Autodesk Fusion 360 part; units mm, degrees
(part 2 of 2)
sketch "Sketch8" plane through (0, 0, -25.2) normal (0, 0, -1) x (1, 0, 0)
  circle A0 centre (107.1093, 9.6234) radius 1.85
  circle A1 centre (13.8605, 220.7337) radius 1.85
  circle A2 centre (13.8605, 111.1767) radius 1.85
  circle A3 centre (13.8605, 9.6234) radius 1.85
  circle A4 centre (107.1093, 220.7337) radius 1.85
  circle A5 centre (106.1086, 111.1767) radius 1.85
  line L0 (118.8791, -2.2165) -> (118.8791, 232.5835)
  line L1 (118.8791, 232.5835) -> (2.0791, 232.5835)
  line L2 (2.0791, 232.5835) -> (2.0791, -2.2165)
  line L3 (2.0791, -2.2165) -> (118.8791, -2.2165)
  circle A6 centre (107.1093, 9.6234) radius 4.65
  circle A7 centre (106.1086, 111.1767) radius 4.65
  circle A8 centre (107.1093, 220.7337) radius 4.65
  line L4 (60.4791, 232.5835) -> (60.4791, -2.2165) construction
  circle A9 centre (13.8605, 111.1767) radius 4.65
  circle A10 centre (13.8605, 220.7337) radius 4.65
  circle A11 centre (13.8605, 9.6234) radius 4.65
  circle A12 centre (107.1093, 220.7337) radius 6.65
  circle A13 centre (13.8605, 220.7337) radius 6.65
  circle A14 centre (106.1086, 111.1767) radius 6.65
  circle A15 centre (13.8605, 111.1767) radius 6.65
  circle A16 centre (13.8605, 9.6234) radius 6.65
  circle A17 centre (107.1093, 9.6234) radius 6.65
  circle A18 centre (13.8605, 9.6234) radius 1.85
  circle A19 centre (13.8605, 111.1767) radius 1.85
  circle A20 centre (107.1093, 220.7337) radius 1.85
  circle A21 centre (106.1086, 111.1767) radius 1.85
  circle A22 centre (13.8605, 220.7337) radius 1.85
  circle A23 centre (107.1093, 9.6234) radius 1.85
  line L5 (111.4791, 5.1835) -> (9.4791, 5.1835)
  line L6 (9.4791, 5.1835) -> (9.4791, 225.1835)
  line L7 (9.4791, 225.1835) -> (111.4791, 225.1835)
  line L8 (111.4791, 225.1835) -> (111.4791, 5.1835)
  line L9 (9.4791, 117.8267) -> (13.8605, 117.8267)
  line L10 (13.8605, 117.8267) -> (13.8605, 104.5267) construction
  line L11 (13.8605, 104.5267) -> (9.4791, 104.5267)
  line L12 (9.4791, 104.5267) -> (9.4791, 117.8267)
  line L13 (111.4791, 117.8267) -> (106.1086, 117.8267)
  line L14 (106.1086, 117.8267) -> (106.1086, 104.5267) construction
  line L15 (106.1086, 104.5267) -> (111.4791, 104.5267)
  line L16 (111.4791, 104.5267) -> (111.4791, 117.8267)
  dimension "d128" = 9.3
  dimension "d129" = 9.3
  dimension "d130" = 9.3
  dimension "d131" = 9.3
  dimension "d132" = 9.3
  dimension "d133" = 9.3
  dimension "d170" = 2
  dimension "d171" = 2
  dimension "d172" = 2
  dimension "d173" = 2
  dimension "d174" = 2
  dimension "d175" = 2
  constraint concentric A0 A6
  constraint concentric A5 A7
  constraint concentric A4 A8
  constraint midpoint L1 L4.start
  constraint midpoint L3 L4.end
  constraint concentric A2 A9
  constraint concentric A1 A10
  constraint concentric A3 A11
  constraint horizontal L9
  constraint vertical L10
  constraint horizontal L11
  constraint vertical L12
  constraint coincident A15 L10.end
  constraint coincident L6 L9.start
  constraint tangent A15 L9
  constraint tangent A15 L11
  constraint horizontal L13
  constraint vertical L14
  constraint horizontal L15
  constraint vertical L16
  constraint coincident A14 L14.end
  constraint coincident L8 L13.start
  constraint tangent A14 L15
  constraint tangent A14 L13
  measures "d128" diameter of A6
  measures "d129" diameter of A7
  measures "d130" diameter of A8
  measures "d131" diameter of A9
  measures "d132" diameter of A10
  measures "d133" diameter of A11
extrude "Extrude17" add sketch "Sketch8" against normal up to surface (6 mm away) contours A6 L8 | A6 A17 L5 L8 | A6 L5 L8 | A6 A17 L5 L8 | A6 L5 L8 | A6 L5 | A14 L8 L15 L16 | A11 A16 L5 L6 | A11 A16 L5 L6 | A14 L8 L16 | A14 L8 L16 | A11 L5 L6 | A11 L5 | A14 L8 L13 L16 | A11 L6 | A15 L6 L11 L12 | A11 L5 L6 | A9 A15 L6 L12 | A9 A15 L6 L12 | A8 A12 L7 L8 | A8 A12 L7 L8 | A15 L6 L9 L12 | A9 L6 L12 | A9 L6 L12 | A8 L8 | A8 L7 L8 | A10 A13 L6 L7 | A10 A13 L6 L7 | A8 L7 | A8 L7 L8 | A10 L7 | A10 L6 L7 | A10 L6 | A10 L6 L7 | A7 bodies 2
extrude "Extrude13" cut sketch "Sketch8" against normal up to surface (3.8 mm away) contours A6 L8 | A6 L5 L8 | A6 L5 | A11 L5 L6 | A11 L5 | A11 L6 | A9 L6 L12 | A9 L6 L12 | A8 L8 | A8 L7 L8 | A8 L7 | A10 L7 | A10 L6 L7 | A10 L6 | A7 picked at (110.6392, 9.6234) picked at (10.3229, 9.6234) picked at (110.6392, 220.7337) picked at (10.3229, 220.7337) bodies 2
fillet "Fillet1" radius 3 16 edges at (2.0791, -232.5835, -8.8) (60.4791, -232.5835, 1.6) (2.0791, -115.1835, 1.6) (118.8791, -232.5835, -8.8) (118.8791, -115.1835, 1.6) (118.8791, 2.2165, -8.8) (60.4791, 2.2165, 1.6) (2.0791, 2.2165, -8.8) (2.0791, -232.5835, -22.2) (2.0791, -115.1835, -25.2) (60.4791, -232.5835, -25.2) (118.8791, -232.5835, -22.2) (118.8791, -115.1835, -25.2) (118.8791, 2.2165, -22.2) (60.4791, 2.2165, -25.2) (2.0791, 2.2165, -22.2) on bodies 1 2
sketch "Sketch9" plane through (0, -232.5835, 0) normal (0, -1, 0) x (1, 0, 0)
  line L0 (115.8791, -1.4) -> (5.0791, -1.4)
  line L1 (5.0791, -1.4) -> (5.0791, -19.2)
  line L2 (46.3791, -23.4) -> (74.5791, -23.4)
  line L3 (5.0791, -25.2) -> (115.8791, -25.2)
  line L4 (60.4791, -1.4) -> (60.4791, -23.6226) construction
  line L5 (46.3791, -12) -> (74.5791, -12)
  line L6 (60.4791, -25.2) -> (60.4791, -23.6226) construction
  line L7 (74.5791, -12) -> (74.5791, -23.4)
  line L8 (46.3791, -23.4) -> (46.3791, -12)
  line L9 (70.9791, -23.4) -> (74.5791, -21.9455)
  line L10 (46.3791, -17.7) -> (74.5791, -17.7) construction
  line L11 (70.9791, -12) -> (74.5791, -13.4545)
  line L12 (49.9791, -23.4) -> (46.3791, -21.9455)
  line L13 (49.9791, -12) -> (46.3791, -13.4545)
  line L14 (115.8791, -19.2) -> (115.8791, -1.4)
  line L15 (5.0791, -19.2) -> (115.8791, -19.2)
  line L16 (72.5791, -12) -> (72.5791, -23.4)
  line L17 (48.3791, -23.4) -> (48.3791, -12)
  line L18 (45.1791, -24.6) -> (75.7791, -24.6)
  line L19 (75.7791, -10.8) -> (75.7791, -24.6)
  line L20 (45.1791, -10.8) -> (75.7791, -10.8)
  line L21 (45.1791, -24.6) -> (45.1791, -10.8)
  line L22 (74.5791, -13.4545) -> (75.7791, -13.4545)
  line L23 (46.3791, -13.4545) -> (45.1791, -13.4545)
  line L24 (74.5791, -13.4545) -> (72.5791, -13.4545)
  line L25 (46.3791, -13.4545) -> (48.3791, -13.4545)
  line L26 (45.1791, -23.4) -> (46.3791, -23.4)
  line L27 (74.5791, -23.4) -> (75.7791, -23.4)
  point P0 (60.4791, -23.4)
  point P1 (60.4791, -12)
  point P2 (60.4791, -17.7)
  point P3 (60.4791, -23.6226)
  point P4 (60.4791, -19.2)
  dimension "d138" = 28.2
  dimension "d139" = 1.8
  dimension "d140" = 28.2
  dimension "d141" = 11.4
  dimension "d143" = 158
  dimension "d144" = 3.6
  dimension "d181" = 2
  dimension "d182" = 2
  dimension "d187" = -1.2
  constraint midpoint L2 P0
  constraint midpoint L0 L4.start
  constraint midpoint L5 P1
  constraint coincident L4 P1
  constraint midpoint L3 L6.start
  constraint coincident P0 L6
  constraint coincident L2 L9.start
  constraint coincident L7 L9.end
  constraint midpoint L8 L10.start
  constraint midpoint L7 L10.end
  constraint symmetric L9.start L10 L11.start
  constraint symmetric L9.end L10 L11.end
  constraint symmetric L4 L9.start L12.start
  constraint symmetric L4 L9.end L12.end
  constraint symmetric L4 L11.start L13.start
  constraint symmetric L4 L11.end L13.end
  constraint midpoint L10 P2
  constraint coincident L4 P2
  constraint coincident P3 L4.end
  constraint midpoint L15 P4
  constraint coincident L4 P4
  constraint coincident L19 L22.end
  constraint perpendicular L19 L22
  constraint coincident L21 L23.end
  constraint perpendicular L21 L23
  constraint coincident L16 L24.end
  constraint perpendicular L16 L24
  constraint coincident L17 L25.end
  constraint perpendicular L17 L25
  constraint coincident L21 L26.start
  constraint perpendicular L8 L26
  constraint coincident L19 L27.end
  constraint perpendicular L19 L27
  measures "d138" distance of L2.start L2.end
  measures "d139" distance of L2 L3
  measures "d140" distance of L5.start L5.end
  measures "d141" distance of L2 L5
  measures "d143" angle of L2 L9
  measures "d144" distance of L2.end L9.start
extrude "Extrude20" add sketch "Sketch9" against normal blind 15.2 from surface at -15 contours L7 L15 L19 L27 | L7 L15 L19 L22 | L8 L15 L21 L23 | L8 L15 L21 L26 | L2 L7 L9 L16 | L2 L8 L12 L17 | L2 L9 L16 | L2 L12 L17 bodies 2
extrude "Extrude14" cut sketch "Sketch9" against normal up to surface (7.4 mm away) contours L7 L15 L16 L24 | L7 L9 L15 L16 | L8 L12 L15 L17 | L8 L15 L17 L25 | L11 L16 L24 | L2 L9 L12 L15 L16 L17 | L5 L11 L13 L15 L16 L17 | L13 L17 L25 bodies 1 2
extrude "Extrude21" add sketch "Sketch9" along normal blind 0.8 from surface at -30.2 contours L7 L15 L16 L24 | L7 L9 L15 L16 | L8 L12 L15 L17 | L8 L15 L17 L25 bodies 2
extrude "Extrude18" add sketch "Sketch9" against normal blind 0.8 contours L7 L9 L15 L16 | L8 L12 L15 L17 bodies 2
extrude "Extrude19" add sketch "Sketch9" against normal blind 0.8 contours L7 L15 L16 L24 | L8 L15 L17 L25 | L11 L16 L24 | L13 L17 L25 bodies 1
fillet "Fillet2" radius 2 4 edges at (46.3791, -228.4835, -13.4545) (74.5791, -228.4835, -13.4545) (46.3791, -228.4835, -21.9455) (74.5791, -228.4835, -21.9455) on bodies 1 2
sketch "Sketch11" plane through (0, -5.1835, 0) normal (0, -1, 0) x (1, 0, 0)
  line L0 (9.4791, -19.2) -> (111.4791, -19.2)
  line L1 (111.4791, -19.2) -> (111.4791, -4.4)
  line L2 (111.4791, -4.4) -> (104.2593, -4.4)
  line L3 (104.2593, -4.4) -> (104.2593, 0)
  line L4 (104.2593, 0) -> (16.6989, 0)
  line L5 (16.6989, 0) -> (16.6989, -4.4)
  line L6 (16.6989, -4.4) -> (9.4791, -4.4)
  line L7 (9.4791, -4.4) -> (9.4791, -19.2)
  line L8 (98.4791, -22.3) -> (89.2791, -22.3)
  line L9 (89.2791, -22.3) -> (89.2791, -16.1)
  line L10 (89.2791, -16.1) -> (98.4791, -16.1)
  line L11 (98.4791, -16.1) -> (98.4791, -22.3)
  line L12 (89.2791, -19.2) -> (98.4791, -19.2) construction
  circle A0 centre (93.8791, -19.2) radius 2.1
  point P0 (98.4791, -19.2)
  dimension "d198" = 6.2
  dimension "d199" = 9.2
  dimension "d200" = 13
  dimension "d201" = 4.2
  constraint horizontal L8
  constraint vertical L9
  constraint horizontal L10
  constraint vertical L11
  constraint midpoint L11 P0
  constraint coincident L0 P0
  constraint midpoint L9 L12.start
  constraint coincident P0 L12.end
  constraint midpoint L12 A0.centre
  measures "d198" distance of L8.start L10.end
  measures "d199" distance of L9 L11
  measures "d200" distance of L1 L11
  measures "d201" diameter of A0
extrude "Extrude22" cut sketch "Sketch11" against normal up to surface (7.4 mm away) contours L0 A0 | L0 A0 bodies 1 2
extrude "Extrude23" cut sketch "Sketch11" against normal up to surface (4 mm away) contours L0 L9 L10 L11 A0 | L0 L8 L9 L11 A0 bodies 1 2
sketch "Sketch12" plane through (0, 0, -23.4) normal (0, 0, 1) x (-1, 0, 0)
  line L0 (-45.1791, 217.5835) -> (-45.1791, 202.3835)
  line L1 (-45.1791, 202.3835) -> (-49.9791, 202.3835)
  line L2 (-49.9791, 202.3835) -> (-49.9791, 217.5835)
  line L3 (-49.9791, 217.5835) -> (-45.1791, 217.5835)
  line L4 (-70.9791, 217.5835) -> (-70.9791, 202.3835)
  line L5 (-70.9791, 202.3835) -> (-75.7791, 202.3835)
  line L6 (-75.7791, 202.3835) -> (-75.7791, 217.5835)
  line L7 (-75.7791, 217.5835) -> (-70.9791, 217.5835)
  arc A0 (-9.4791, 14.626) -> (-18.8113, 5.1835) centre (-13.8605, 9.6234) ccw
  line L8 (-9.4791, 14.626) -> (-9.4791, 104.5267)
  line L9 (-9.4791, 104.5267) -> (-13.8605, 104.5267)
  arc A1 (-13.8605, 117.8267) -> (-13.8605, 104.5267) centre (-13.8605, 111.1767) ccw
  line L10 (-13.8605, 117.8267) -> (-9.4791, 117.8267)
  line L11 (-9.4791, 117.8267) -> (-9.4791, 215.7311)
  arc A2 (-18.8024, 225.1835) -> (-9.4791, 215.7311) centre (-13.8605, 220.7337) ccw
  line L12 (-18.8024, 225.1835) -> (-49.9791, 225.1835)
  line L13 (-49.9791, 225.1835) -> (-49.9791, 232.333)
  line L14 (-49.9791, 232.333) -> (-70.9791, 232.333)
  line L15 (-70.9791, 232.333) -> (-70.9791, 225.1835)
  line L16 (-70.9791, 225.1835) -> (-102.1674, 225.1835)
  arc A3 (-111.4791, 215.721) -> (-102.1674, 225.1835) centre (-107.1093, 220.7337) ccw
  line L17 (-111.4791, 215.721) -> (-111.4791, 117.8267)
  line L18 (-111.4791, 117.8267) -> (-106.1086, 117.8267)
  arc A4 (-106.1086, 104.5267) -> (-106.1086, 117.8267) centre (-106.1086, 111.1767) ccw
  line L19 (-106.1086, 104.5267) -> (-111.4791, 104.5267)
  line L20 (-111.4791, 104.5267) -> (-111.4791, 14.6361)
  arc A5 (-102.1585, 5.1835) -> (-111.4791, 14.6361) centre (-107.1093, 9.6234) ccw
  line L21 (-102.1585, 5.1835) -> (-18.8113, 5.1835)
  line L22 (-89.2791, 1.1835) -> (-98.4791, 1.1835)
  line L23 (-89.2791, 5.7835) -> (-98.4791, 5.7835)
  line L24 (-95.0791, 5.7835) -> (-92.6791, 5.7835)
  line L25 (-92.6791, 5.7835) -> (-92.6791, 10.1835)
  line L26 (-92.6791, 10.1835) -> (-95.0791, 10.1835)
  line L27 (-95.0791, 10.1835) -> (-95.0791, 5.7835)
  point P0 (-93.8791, 5.7835)
  point P1 (-93.8791, 5.7835)
  dimension "d206" = 4.6
  dimension "d207" = 2.4
  dimension "d208" = 4.4
  constraint horizontal L24
  constraint vertical L25
  constraint horizontal L26
  constraint vertical L27
  constraint coincident L23 L24.start
  constraint midpoint L23 P1
  constraint midpoint L24 P1
  constraint coincident P1 P0
  measures "d207" distance of L24.start L24.end
  measures "d208" distance of L24.start L26.end
extrude "Extrude24" add sketch "Sketch12" along normal up to surface (6.3 mm away) contours L23 L24 L25 L26 L27 bodies 2
sketch "Sketch10" plane through (0, -5.1835, 0) normal (0, -1, 0) x (1, 0, 0)
  line L0 (16.6989, -4.4) -> (9.4791, -4.4)
  line L1 (9.4791, -4.4) -> (9.4791, -19.2)
  line L2 (111.4791, -19.2) -> (111.4791, -4.4)
  line L3 (104.2593, -4.4) -> (104.2593, 0)
  line L4 (104.2593, 0) -> (16.6989, 0)
  line L5 (16.6989, 0) -> (16.6989, -4.4)
  line L6 (19.0989, -19.8) -> (34.8989, -19.8)
  line L7 (34.8989, -19.8) -> (34.8989, -18.6)
  line L8 (34.8989, -18.6) -> (19.0989, -18.6)
  line L9 (19.0989, -18.6) -> (19.0989, -19.8)
  line L10 (26.9989, -19.8) -> (26.9989, -18.6) construction
  line L11 (30.4989, -17.6) -> (23.4989, -17.6)
  arc A0 (23.4989, -17.6) -> (23.4989, -20.8) centre (23.4989, -19.2) ccw
  line L12 (23.4989, -20.8) -> (30.4989, -20.8)
  arc A1 (30.4989, -20.8) -> (30.4989, -17.6) centre (30.4989, -19.2) ccw
  line L13 (30.4989, -19.2) -> (23.4989, -19.2) construction
  line L14 (98.4791, -19.2) -> (111.4791, -19.2)
  line L15 (111.4791, -4.4) -> (104.2593, -4.4)
  line L16 (98.4791, -16.1) -> (98.4791, -19.2)
  line L17 (9.4791, -19.2) -> (89.2791, -19.2)
  line L18 (89.2791, -19.2) -> (89.2791, -16.1)
  line L19 (89.2791, -16.1) -> (98.4791, -16.1)
  point P0 (26.9989, -19.2)
  dimension "d160" = 15.8
  dimension "d161" = 1.2
  dimension "d162" = 2.4
  dimension "d163" = 3.5
  dimension "d164" = 3.2
  constraint horizontal L6
  constraint vertical L7
  constraint horizontal L8
  constraint vertical L9
  constraint midpoint L6 L10.start
  constraint midpoint L8 L10.end
  constraint tangent L11 A0
  constraint tangent A0 L12
  constraint parallel L11 L12
  constraint tangent L12 A1
  constraint tangent L11 A1
  constraint perpendicular L10 L13
  constraint midpoint L10 P0
  constraint midpoint L13 P0
  constraint coincident A1.centre L14
  measures "d160" distance of L6.start L6.end
  measures "d161" distance of L6.start L8.end
  measures "d162" distance of L5 L9
  measures "d163" distance of A0.centre P0
  measures "d164" diameter of A0
extrude "Extrude16" cut sketch "Sketch10" against normal up to surface (5.8 mm away) contours L6 L9 A0 L17 | L8 L9 A0 L17 | L6 L7 A1 L17 | L7 L8 A1 L17 bodies 1
extrude "Extrude15" cut sketch "Sketch10" against normal up to surface (7.4 mm away) contours L6 A0 A1 L17 | L8 A0 A1 L17 | L8 L11 A0 A1 | L6 A0 L12 A1 bodies 1 2
sketch "Sketch13" plane through (0, 0, -23.4) normal (0, 0, 1) x (-1, 0, 0)
  line L0 (-95.0791, 5.7835) -> (-95.0791, 10.1835)
  line L1 (-95.0791, 10.1835) -> (-92.6791, 10.1835)
  line L2 (-92.6791, 10.1835) -> (-92.6791, 5.7835)
  line L3 (-92.6791, 5.7835) -> (-95.0791, 5.7835)
  line L4 (-45.1791, 217.5835) -> (-45.1791, 202.3835)
  line L5 (-45.1791, 202.3835) -> (-49.9791, 202.3835)
  line L6 (-49.9791, 202.3835) -> (-49.9791, 217.5835)
  line L7 (-49.9791, 217.5835) -> (-45.1791, 217.5835)
  line L8 (-70.9791, 217.5835) -> (-70.9791, 202.3835)
  line L9 (-70.9791, 202.3835) -> (-75.7791, 202.3835)
  line L10 (-75.7791, 202.3835) -> (-75.7791, 217.5835)
  line L11 (-75.7791, 217.5835) -> (-70.9791, 217.5835)
  arc A0 (-9.4791, 14.626) -> (-18.8113, 5.1835) centre (-13.8605, 9.6234) ccw
  line L12 (-9.4791, 14.626) -> (-9.4791, 104.5267)
  line L13 (-9.4791, 104.5267) -> (-13.8605, 104.5267)
  arc A1 (-13.8605, 117.8267) -> (-13.8605, 104.5267) centre (-13.8605, 111.1767) ccw
  line L14 (-13.8605, 117.8267) -> (-9.4791, 117.8267)
  line L15 (-9.4791, 117.8267) -> (-9.4791, 215.7311)
  arc A2 (-18.8024, 225.1835) -> (-9.4791, 215.7311) centre (-13.8605, 220.7337) ccw
  line L16 (-18.8024, 225.1835) -> (-49.9791, 225.1835)
  line L17 (-49.9791, 225.1835) -> (-49.9791, 232.333)
  line L18 (-49.9791, 232.333) -> (-70.9791, 232.333)
  line L19 (-70.9791, 232.333) -> (-70.9791, 225.1835)
  line L20 (-70.9791, 225.1835) -> (-102.1674, 225.1835)
  arc A3 (-111.4791, 215.721) -> (-102.1674, 225.1835) centre (-107.1093, 220.7337) ccw
  line L21 (-111.4791, 215.721) -> (-111.4791, 117.8267)
  line L22 (-111.4791, 117.8267) -> (-106.1086, 117.8267)
  arc A4 (-106.1086, 104.5267) -> (-106.1086, 117.8267) centre (-106.1086, 111.1767) ccw
  line L23 (-106.1086, 104.5267) -> (-111.4791, 104.5267)
  line L24 (-111.4791, 104.5267) -> (-111.4791, 14.6361)
  arc A5 (-102.1585, 5.1835) -> (-111.4791, 14.6361) centre (-107.1093, 9.6234) ccw
  line L25 (-102.1585, 5.1835) -> (-18.8113, 5.1835)
  line L26 (-22.0157, 14.3835) -> (-19.0989, 14.3835)
  line L27 (-19.0989, 5.1835) -> (-22.0157, 5.1835)
  line L28 (-19.0989, 5.1835) -> (-19.0989, 14.3835)
  line L29 (-22.0157, 5.1835) -> (-22.0157, 14.3835)
  line L30 (-19.0989, 14.3835) -> (-21.4157, 14.3835)
  line L31 (-21.4157, 14.3835) -> (-21.4157, 20.3835)
  line L32 (-21.4157, 20.3835) -> (-19.0989, 20.3835)
  line L33 (-19.0989, 20.3835) -> (-19.0989, 14.3835)
  line L34 (-19.0989, 14.3835) -> (-21.4157, 14.3835)
  line L35 (-21.4157, 14.3835) -> (-21.4157, 10.3835)
  line L36 (-21.4157, 10.3835) -> (-19.0989, 10.3835)
  line L37 (-19.0989, 10.3835) -> (-19.0989, 14.3835)
  dimension "d211" = 9.2
  dimension "d212" = 90
  dimension "d213" = 6
  dimension "d214" = 0.6
  dimension "d217" = 4
  constraint parallel L25 L26
  constraint coincident L27.start L28.start
  constraint coincident L27.end L29.start
  constraint coincident L26 L29.end
  constraint perpendicular L26 L29
  constraint coincident L26.start L29
  constraint horizontal L30
  constraint vertical L31
  constraint horizontal L32
  constraint vertical L33
  constraint perpendicular L34 L35
  constraint parallel L34 L36
  constraint parallel L35 L37
  measures "d211" distance of L25 L26
  measures "d212" angle of L26 L28
  measures "d213" distance of L26.end L32.end
  measures "d214" distance of L29 L31
  measures "d217" distance of L26.end L36.end
extrude "Extrude25" add sketch "Sketch13" along normal up to surface (6.2 mm away) contours L26 L30 L31 L32 L33 L34 bodies 2
chamfer "Chamfer1" distance 5.6 angle 45 1 edges at (20.2573, -20.3835, -23.4) on bodies 2
extrude "Extrude26" add sketch "Sketch13" along normal up to surface (4.2 mm away) contours A0 L26 L28 L30 L34 L35 L36 L37 bodies 2
equation "ledHoleDistance = 8.1 mm"
equation "ledHoleDiameter = 7 mm"
equation "d28 = ledHoleDistance"
equation "d29 = ledHoleDistance"
equation "d30 = ledHoleDistance"
equation "d31 = ledHoleDistance"
equation "d35 = ledHoleDistance"
equation "d36 = ledHoleDistance"
equation "d37 = ledHoleDistance"
equation "d38 = ledHoleDistance"
equation "d39 = ledHoleDistance"
equation "d40 = ledHoleDistance"
equation "d44 = ledHoleDiameter"
equation "d45 = ledHoleDiameter"
equation "d46 = ledHoleDiameter"
equation "d47 = ledHoleDiameter"
equation "d48 = ledHoleDiameter"
equation "d49 = ledHoleDiameter"
equation "d50 = ledHoleDiameter"
equation "d51 = ledHoleDiameter"
equation "d52 = ledHoleDiameter"
equation "d53 = ledHoleDiameter"
equation "d54 = topThickness"
equation "d56 = screwHoleDiameter"
equation "screwHoleDiameter = 3.7 mm"
equation "d58 = screwHoleDiameter"
equation "d59 = screwHoleDiameter"
equation "d60 = screwHoleDiameter"
equation "d61 = screwHoleDiameter"
equation "d62 = screwHoleDiameter"
equation "topThickness = 1.6 mm"
equation "topFromPCBDistance = 4.4 mm"
equation "d75 = -topFromPCBDistance"
equation "pcbWidth = 102 mm"
equation "pcbLength = 220 mm"
equation "d79 = pcbWidth"
equation "d80 = pcbLength"
equation "d81 = ledStripSupportWallWidth"
equation "d82 = -( topFromPCBDistance + pcbThickness + ledStripWidth )"
equation "spaceUnderPcb = 17.2 mm"
equation "ledStripWidth = 13 mm"
equation "bottomThickness = 1.8 mm"
equation "pcbThickness = 1.8 mm"
equation "ledStripThickness = 3.4 mm"
equation "d89 = ledStripSupportWallWidth + ledStripThickness"
equation "ledStripDiffusionSpace = 2.4 mm"
equation "d93 = ledStripSupportWallWidth + ledStripThickness + ledStripDiffusionSpace"
equation "d97 = -( topFromPCBDistance + pcbThickness )"
equation "d99 = ledStripThickness * 2"
equation "d102 = ledStripThickness"
equation "d103 = ledStripWidth"
equation "d105 = ledStripThickness"
equation "d106 = ledStripThickness"
equation "d112 = screwHoleDiameter / 2 + 1 mm"
equation "d113 = screwHoleDiameter / 2 + 1 mm"
equation "d114 = screwHoleDiameter / 2 + 1 mm"
equation "d115 = screwHoleDiameter / 2 + 1 mm"
equation "d116 = spaceUnderPcb - ledStripWidth"
equation "d118 = bottomThickness"
equation "d128 = bottomNutSlotWidth"
equation "d129 = bottomNutSlotWidth"
equation "d130 = bottomNutSlotWidth"
equation "d131 = bottomNutSlotWidth"
equation "d132 = bottomNutSlotWidth"
equation "d133 = bottomNutSlotWidth"
equation "d139 = bottomThickness"
equation "bottomNutSlotWidth = 9.3 mm"
equation "ledStripSupportWallWidth = 1.6 mm"
equation "d190 = -14.4 mm - 0.8 mm"
equation "sideButtonHeight = 6.2 mm"
equation "d198 = sideButtonHeight"
named bodies: "top", "bottom"
